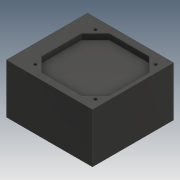
# Autodesk Inventor part: 파워서플라이
Saved by Autodesk Inventor 2018 (Build 220112000, 112)
## iProperties
Created: 2018-10-27
Part Number: 파워서플라이
Material: 일반
Document SubType Name: Modeling
Designer: dhksr
Density: 1 g/cm^3
Appearance: 매끄러움 - 검은색
Author: dhksr
Autodesk Inventor part; units mm, degrees
ref_plane "YZ Plane" through (0, 0, 0) normal (1, 0, 0) x (0, 1, 0)
ref_plane "XZ Plane" through (0, 0, 0) normal (0, 1, 0) x (-1, 0, 0)
ref_plane "XY Plane" through (0, 0, 0) normal (0, 0, 1) x (1, 0, 0)
sketch "스케치1" plane through (0, 0, 0) normal (0, 0, 1) x (1, 0, 0)
  line L0 (0, 0) -> (150, 0)
  line L1 (150, 0) -> (150, 141.5)
  line L2 (150, 141.5) -> (0, 141.5)
  line L3 (0, 141.5) -> (0, 0)
  dimension "d0" = 150
  dimension "d1" = 141.5
  constraints: 8 end point, 2 parallel, 1 horizontal, 1 perpendicular
  measures "d0" distance of L2.end L1.end
  measures "d1" distance of L1.end L0.end
extrude "돌출1" add sketch "스케치1" along normal blind 86.5
sketch "스케치2" plane through (0, 0, 86.5) normal (0, 0, 1) x (1, 0, 0)
  line L0 (150, 0) -> (150, 141.5) projected
  line L1 (137, 18.25) -> (32, 18.25) construction
  line L2 (32, 18.25) -> (32, 123.25) construction
  line L3 (32, 123.25) -> (137, 123.25) construction
  line L4 (137, 123.25) -> (137, 18.25) construction
  line L5 (137, 18.25) -> (32, 123.25) construction
  line L6 (32, 18.25) -> (137, 123.25) construction
  circle A0 centre (32, 123.25) radius 2.5
  circle A1 centre (32, 18.25) radius 2.5
  circle A2 centre (137, 18.25) radius 2.5
  circle A3 centre (137, 123.25) radius 2.5
  point P0 (84.5, 70.75)
  point P1 (32, 70.75)
  point P2 (0, 70.75)
  dimension "d4" = 105
  dimension "d5" = 105
  dimension "d7" = 13
  dimension "d9" = 5
  dimension "d12" = 360
  constraints: 12 end point, 4 centre point, 3 midpoint, 2 parallel, 1 coincident, 1 horizontal, 1 horizontal alignment, 1 perpendicular, 9 other
  measures "d4" distance of L1.end L2.end
  measures "d5" distance of L2.end L3.end
  measures "d7" distance between parallel lines of L0 L4
  measures "d9" diameter of A0
extrude "돌출2" cut sketch "스케치2" against normal blind 5
sketch "스케치3" plane through (0, 0, 86.5) normal (0, 0, 1) x (1, 0, 0)
  circle A0 centre (32, 123.25) radius 2.5 construction
  circle A1 centre (137, 18.25) radius 2.5 construction
  line L0 (32, 123.25) -> (137, 123.25) construction
  line L1 (137, 123.25) -> (137, 18.25) construction
  line L2 (137, 18.25) -> (32, 18.25) construction
  line L3 (32, 18.25) -> (32, 123.25) construction
  line L4 (84.5, 123.25) -> (84.5, 70.75) construction
  line L5 (84.5, 70.75) -> (137, 70.75) construction
  line L6 (119.3236, 11.75) -> (49.6764, 11.75)
  line L7 (25.5, 35.9264) -> (25.5, 105.5736)
  line L8 (49.6764, 129.75) -> (119.3236, 129.75)
  line L9 (143.5, 105.5736) -> (143.5, 35.9264)
  line L10 (143.5, 11.75) -> (25.5, 129.75) construction
  line L11 (25.5, 11.75) -> (143.5, 129.75) construction
  line L12 (119.3236, 129.75) -> (143.5, 105.5736)
  line L13 (25.5, 105.5736) -> (49.6764, 129.75)
  line L14 (49.6764, 11.75) -> (25.5, 35.9264)
  line L15 (143.5, 35.9264) -> (119.3236, 11.75)
  point P0 (150, 141.5)
  dimension "d28" = 360
  dimension "d16" = 90
  dimension "d21" = 118
  dimension "d22" = 45
  dimension "d24" = 45
  dimension "d25" = 30
  constraints: 32 end point, 4 parallel, 3 midpoint, 2 horizontal, 2 perpendicular, 1 vertical, 13 other
  measures "d16" angle of L5 L4
  measures "d21" distance of L10.end L11.end
  measures "d22" angle of L8 L10
  measures "d24" angle of L9 L12
  measures "d25" distance from line of point (150, 141.5) L12
extrude "돌출3" cut sketch "스케치3" against normal blind 10
sketch "스케치4" plane through (0, 141.5, 0) normal (0, 1, 0) x (1, 0, 0)
  line L0 (20.5008, -63.1326) -> (20.5008, -47.8147)
  line L1 (20.5008, -47.8147) -> (50.8737, -47.8147)
  line L2 (50.8737, -47.8147) -> (50.8737, -63.1326)
  line L3 (50.8737, -63.1326) -> (42.1805, -66.6205)
  line L4 (42.1805, -66.6205) -> (29.194, -66.6205)
  line L5 (29.194, -66.6205) -> (20.5008, -63.1326)
  point P0 (35.6872, -66.6205)
  point P1 (35.6872, -47.8147)
  constraints: 12 end point, 2 horizontal, 2 midpoint, 1 horizontal alignment, 1 parallel, 1 vertical, 1 vertical alignment
extrude "돌출4" cut sketch "스케치4" against normal blind 10
